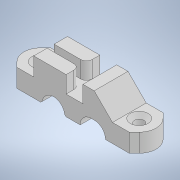
# Autodesk Inventor part: Magnet Mount Lower
Saved by Autodesk Inventor 2022 (Build 260153000, 153)
## iProperties
Created: 2022-04-23
Part Number: Magnet Mount Lower
Material: Generic
Document SubType Name: Modeling
Designer: Nick
Density: 1 g/cm^3
Appearance: Default
Author: Nick
Autodesk Inventor part; units mm, degrees
ref_plane "YZ Plane" through (0, 0, 0) normal (1, 0, 0) x (0, 1, 0)
ref_plane "XZ Plane" through (0, 0, 0) normal (0, 1, 0) x (-1, 0, 0)
ref_plane "XY Plane" through (0, 0, 0) normal (0, 0, 1) x (1, 0, 0)
sketch "Sketch1" plane through (0, 0, 0) normal (0, 0, 1) x (1, 0, 0)
  line L0 (0, 0) -> (28, 0)
  line L1 (28, 0) -> (28, 13)
  line L2 (28, 13) -> (0, 13)
  line L3 (0, 13) -> (0, 0)
  circle A0 centre (7, 0) radius 4
  circle A1 centre (21, 0) radius 4 construction
  line L4 (21, 0) -> (23, 0) construction
  line L5 (20.5, 0) -> (21.5, 0) construction
  line L6 (20.5, 4) -> (21.5, 4)
  line L7 (21.5, -4) -> (20.5, -4)
  arc A2 (20.5, 4) -> (20.5, -4) centre (20.5, 0) ccw
  arc A3 (21.5, -4) -> (21.5, 4) centre (21.5, 0) ccw
  point P0 (3, 0)
  point P1 (11, 0)
  point P2 (17, 0)
  point P3 (25, 0)
  point P4 (22, 0)
  point P5 (21, 0)
  point P6 (16.5, 0)
  point P7 (25.5, 0)
  dimension "d0" = 28
  dimension "d1" = 13
  dimension "d2" = 8
  dimension "d3" = 8
  dimension "d4" = 14
  dimension "d5" = 7
  dimension "d6" = 7
  dimension "d39" = 1
  dimension "d40" = 1
  constraints: 20 end point, 4 centre point, 4 point on circle, 4 tangent, 3 parallel, 3 point on line, 2 horizontal, 2 midpoint, 1 coincident, 1 equal radius, 1 perpendicular
  measures "d0" distance of L1.end L2.end
  measures "d1" distance of L0.end L1.end
  measures "d2" diameter of A0
  measures "d3" diameter of A1
  measures "d4" distance of L4.start A0.centre
  measures "d5" distance from line of L1 L4.start
  measures "d6" distance from line of A0.centre L3
  measures "d39" distance of L4.start point (22, 0)
  measures "d40" distance of L5.end L5.start
extrude "Extrusion1" add sketch "Sketch1" along normal blind 12 contours L3 L2 L1 L0 A3 L6 A2 A0
chamfer "Chamfer1" distance 6.5 angle 45 1 edges at (28, 13, 6)
sketch "Sketch2" plane through (0, 13, 12) normal (0, 1, 0) x (1, 0, 0)
  line L0 (0, 12) -> (0, 0) projected
  line L1 (0, 7.25) -> (11.5, 7.25)
  line L2 (11.5, 7.25) -> (11.5, 12)
  line L3 (21.5, 12) -> (0, 12) projected
  line L4 (17.5, 12) -> (17.5, 0)
  line L5 (11, 0) -> (3, 0) projected
  line L6 (0, 4.75) -> (11.5, 4.75)
  line L7 (11.5, 4.75) -> (11.5, 0)
  line L8 (11, 0) -> (3, 0) projected
  line L9 (11.5, 12) -> (17.5, 12)
  line L10 (17.5, 0) -> (11.5, 0)
  line L11 (0, 4.75) -> (0, 7.25)
  point P0 (17, 0)
  dimension "d12" = 6
  dimension "d13" = 2.5
  dimension "d14" = 11.5
  constraints: 16 end point, 6 point on line, 3 perpendicular, 2 collinear, 2 horizontal, 1 vertical
  measures "d12" distance between parallel lines of L4 L2
  measures "d13" distance between parallel lines of L6 L1
  measures "d14" distance of L1.start L1.end
extrude "Extrusion2" cut sketch "Sketch2" against normal blind 6 contours L1 L2 L3 L4 L10 L7 L6 L0
fillet "Fillet1" radius 2 2 edges at (11.5, 10, 4.75) (11.5, 10, 7.25)
chamfer "Chamfer2" distance 0.5 angle 45 2 edges at (3, 0, 6) (11, 0, 6)
ref_plane "Work Plane1" through (0, 0, 6) normal (0, 0, 1) x (1, 0, 0)
ref_plane "Work Plane3" through (14, 0, 12) normal (1, 0, 0) x (0, 0, -1)
sketch "Sketch5" plane through (28, 0, 0) normal (0, -1, 0) x (1, 0, 0)
  circle A0 centre (3.5, 6) radius 1.5
  line L0 (-28, 0) -> (-25.5, 0) projected
  line L1 (0, 0) -> (0, 12) projected
  circle A1 centre (3.5, 6) radius 3.5
  line L2 (0, 0) -> (0, 12) projected
  line L3 (-6.5, 12) -> (0, 12) projected
  line L4 (0, 12) -> (5.9853, 12)
  line L5 (0, 0) -> (-6.5, 0) projected
  line L6 (0, 0) -> (5.9853, 0)
  line L7 (5.9853, 0) -> (7.7426, 1.7574)
  line L8 (5.9853, 12) -> (7.7426, 10.2426)
  circle A2 centre (3.5, 6) radius 6
  line L9 (-28, 12) -> (-25.5, 12) projected
  line L10 (-28, 0) -> (-28, 12) projected
  line L11 (-25.5, 12) -> (-25.5, 0) projected
  line L12 (-16.5, 0) -> (-16.5, 12) projected
  line L13 (-16.5, 0) -> (-11.5, 0) projected
  line L14 (-11.5, 0) -> (-11.5, 12) projected
  line L15 (-16.5, 12) -> (-11.5, 12) projected
  line L16 (-2.5, 0) -> (0, 0) projected
  line L17 (-2.5, 12) -> (0, 12) projected
  line L18 (-2.5, 0) -> (-2.5, 12) projected
  point P0 (0, 6)
  dimension "d26" = 3
  dimension "d28" = 7
  dimension "d38" = 135
  constraints: 8 end point, 4 tangent, 3 centre point, 2 coincident, 2 equal length, 2 horizontal, 2 point on circle, 1 horizontal alignment, 1 midpoint
  measures "d26" diameter of A0
  measures "d28" diameter of A1
  measures "d38" angle of L6 L7
extrude "Extrusion3" add sketch "Sketch5" against normal blind 6.5 contours A0 | L1 A2 L6 | A1 | L1 A2 | A2 L7 L6 | L1 L4 A2 | L4 L8 A2 picked at (0.8638, 10.4147)
sketch "Sketch6" plane through (28, 6.5, 0) normal (0, 1, 0) x (1, 0, 0)
  arc A0 (7.7426, -10.2426) -> (7.7426, -1.7574) centre (3.5, -6) ccw projected
  point P0 (-28, 0)
hole "Hole1" at (31.5, 6.5, 6) direction (0, -1, 0) diameter 3.4 depth 8 countersink diameter 6.3 countersink angle 90 clearance for "Flat Head Machine Screw" size "M3" standard "Ansi Metric M Profile"
mirror "Mirror2" about plane through (14, 0, 12) normal (1, 0, 0) of "Extrusion3", "Hole1"
equation "\"d5\" = d6"
body "Solid1"
